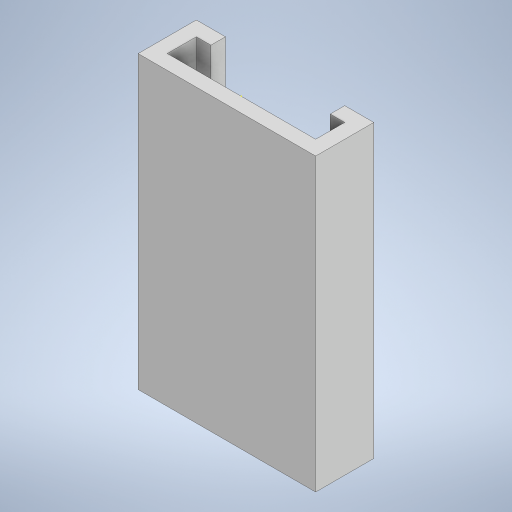
# Autodesk Inventor part: wsb
Saved by Autodesk Inventor 2024.1 (Build 281209000, 209)
## iProperties
Created: 2024-10-07
Part Number: wsb
Material: Všeobecné
Document SubType Name: Modeling
Designer: elias
Density: 1 g/cm^3
Appearance: Výchozí
Author: elias
Autodesk Inventor part; units mm, degrees
ref_plane "YZ Plane" through (0, 0, 0) normal (1, 0, 0) x (0, 1, 0)
ref_plane "XZ Plane" through (0, 0, 0) normal (0, 1, 0) x (-1, 0, 0)
ref_plane "XY Plane" through (0, 0, 0) normal (0, 0, 1) x (1, 0, 0)
sketch "Náčrt1" plane through (0, 0, 0) normal (0, 0, 1) x (1, 0, 0)
  line L0 (0, 0) -> (5.1, 0)
  line L1 (5.1, 0) -> (5.1, 2)
  line L2 (5.1, 2) -> (4.1, 2)
  line L3 (4.1, 2) -> (4.1, 3)
  line L4 (4.1, 3) -> (6.1, 3)
  line L5 (6.1, 3) -> (6.1, 0)
  line L6 (6.1, 0) -> (6.1, -1)
  line L7 (6.1, -1) -> (0, -1)
  line L8 (0, 0) -> (0, -1)
  line L9 (0, 0) -> (-5.1, 0)
  line L10 (-5.1, 0) -> (-5.1, 2)
  line L11 (-5.1, 2) -> (-4.1, 2)
  line L12 (-4.1, 2) -> (-4.1, 3)
  line L13 (-4.1, 3) -> (-6.1, 3)
  line L14 (-6.1, 3) -> (-6.1, 0)
  line L15 (-6.1, 0) -> (-6.1, -1)
  line L16 (-6.1, -1) -> (0, -1)
  point P0 (4.1, 2)
  point P1 (-4.1, 2)
  dimension "d0" = 5.1
  dimension "d1" = 2
  dimension "d2" = 1
  dimension "d3" = 1
  dimension "d4" = 2
  dimension "d5" = 1
  constraints: 34 end point, 8 symmetric about line, 4 perpendicular, 3 horizontal, 2 point on line, 1 vertical
  measures "d0" distance of L0.start L0.end
  measures "d1" distance of L0.end L1.end
  measures "d2" distance of L1.end L2.end
  measures "d3" distance of L2.end L3.end
  measures "d4" distance of L3.end L4.end
  measures "d5" distance of L5.end L6.end
extrude "Vysunutí1" add sketch "Náčrt1" along normal blind 20
sketch "Náčrt2" plane through (0, 0, 20) normal (0, 0, 1) x (1, 0, 0)
  point P0 (0, 0)
